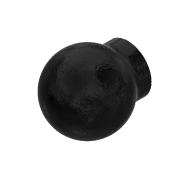
# Autodesk Inventor part: endEffector
Saved by Autodesk Inventor 2021 (Build 250183000, 183)
## iProperties
Created: 2020-08-17
Part Number: endEffector
Material: Generic
Document SubType Name: Modeling
Designer: Derm
Density: 1 g/cm^3
Appearance: Fine Textured - Black
Author: Derm
Autodesk Inventor part; units mm, degrees
ref_plane "YZ Plane" through (0, 0, 0) normal (1, 0, 0) x (0, 1, 0)
ref_plane "XZ Plane" through (0, 0, 0) normal (0, 1, 0) x (-1, 0, 0)
ref_plane "XY Plane" through (0, 0, 0) normal (0, 0, 1) x (1, 0, 0)
sketch "Sketch1" plane through (0, 0, 0) normal (0, 0, 1) x (1, 0, 0)
  circle A0 centre (0, 0) radius 25.56 projected
  point P0 (0, 0)
extrude "Extrusion1" add sketch "Sketch1" along normal blind 15.9004
sketch "Sketch2" plane through (0, 0, 0) normal (1, 0, 0) x (0, 1, 0)
  line L0 (25.56, 0) -> (25.56, 15.9004) projected
  line L1 (0, 0) -> (0, 82.2545)
  arc A0 (25.56, 15.9004) -> (0, 82.2545) centre (0, 44.1545) ccw
  line L2 (25.56, 15.9004) -> (0, 15.9004)
  line L3 (25.56, 15.9004) -> (-25.56, 15.9004) projected
  point P0 (0, 15.9004)
  dimension "d3" = 38.1
  constraints: 4 end point, 2 point on circle, 1 centre point, 1 midpoint, 1 point on line, 1 vertical
  measures "d3" radius of A0
revolve "Revolution1" add sketch "Sketch2" angle 360 about axis through (0, 0, 0) along (0, 0, 1)
fillet "Fillet1" radius 12.7 2 edges at (-18.0737, -18.0737, 15.9004) (18.0737, 18.0737, 15.9004)
body "Solid1"
